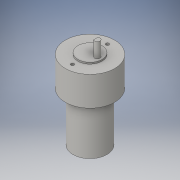
# Autodesk Inventor part: Autofeeder motor
Saved by Autodesk Inventor 2016 (Build 200138000, 138)
## iProperties
Created: 2016-12-12
Part Number: Autofeeder motor
Material: Generic
Document SubType Name: Modeling
Designer: Student
Density: 1 g/cm^3
Appearance: Default
Author: Student
Autodesk Inventor part; units mm, degrees
ref_plane "YZ Plane" through (0, 0, 0) normal (1, 0, 0) x (0, 1, 0)
ref_plane "XZ Plane" through (0, 0, 0) normal (0, 1, 0) x (-1, 0, 0)
ref_plane "XY Plane" through (0, 0, 0) normal (0, 0, 1) x (1, 0, 0)
sketch "Sketch1" plane through (0, 0, 0) normal (0, 1, 0) x (-1, 0, 0)
  circle A0 centre (0, 0) radius 20.1549
  dimension "d0" = 40.3098
  constraints: 1 centre point, 1 coincident
  measures "d0" diameter of A0
extrude "Extrusion1" add sketch "Sketch1" along normal blind 58.2676
sketch "Sketch2" plane through (0, 58.2676, 0) normal (0, 1, 0) x (1, 0, 0)
  circle A0 centre (0, 0) radius 29.21
  dimension "d3" = 58.42
  constraints: 1 centre point, 1 coincident
  measures "d3" diameter of A0
extrude "Extrusion2" add sketch "Sketch2" along normal blind 34.7726
sketch "Sketch3" plane through (0, 93.0402, 0) normal (0, 1, 0) x (1, 0, 0)
  circle A0 centre (0, 0) radius 14.3002
  dimension "d6" = 28.6004
  constraints: 1 centre point, 1 coincident
  measures "d6" diameter of A0
extrude "Extrusion3" add sketch "Sketch3" along normal blind 1.8288
sketch "Sketch4" plane through (0, 93.0402, 0) normal (0, 1, 0) x (1, 0, 0)
  circle A0 centre (0, 20.7518) radius 1.905
  circle A1 centre (0, 0) radius 14.3002 projected
  line L0 (-34.2978, 0) -> (34.9424, 0) construction
  circle A2 centre (0, -20.7518) radius 1.905
  dimension "d9" = 3.81
  dimension "d10" = 4.5466
  constraints: 2 centre point, 2 end point, 1 horizontal, 1 symmetric about line, 1 other
  measures "d9" diameter of A0
extrude "Extrusion4" cut sketch "Sketch4" against normal blind 33.02 contours A0 | A2
sketch "Sketch5" plane through (0, 94.869, 0) normal (0, 1, 0) x (1, 0, 0)
  circle A0 centre (8.6926, 0) radius 3.1877
  point P0 (0, 0)
  dimension "d13" = 6.3754
  dimension "d14" = 8.6926
  constraints: 1 centre point
  measures "d13" diameter of A0
  measures "d14" distance of point (0, 0) A0.centre
extrude "Extrusion5" add sketch "Sketch5" along normal blind 17.78
sketch "Sketch6" plane through (8.6926, 112.649, 0) normal (0, 1, 0) x (1, 0, 0)
  circle A0 centre (0, 0) radius 3.1877 projected
  line L0 (-1.8509, -2.5953) -> (-1.8509, 2.5953)
  arc A1 (-1.8509, 2.5953) -> (-1.8509, -2.5953) centre (0, 0) ccw
  point P0 (-8.6926, 0)
  constraints: 4 point on circle, 2 end point, 1 centre point, 1 concentric, 1 vertical
extrude "Extrusion6" cut sketch "Sketch6" against normal blind 17.78 contours L0 A0 picked at (-2.2965, 0)
body "Solid1"
